Decora_1-Gang_v4 (Autodesk Fusion 360 design; units mm, degrees)
Autodesk Fusion 360 part; units mm, degrees
note: some values were not read from the file. Chosen so that the rebuilt part matches the saved one: which bodies a step acts on; which face or edge a step refers to; which pieces of a blend or face edit are solid. Set by a fixed rule: which sketch regions a step uses.
sketch "Sketch1" plane through (0, 0, 0) normal (0, 0, 1) x (1, 0, 0)
  line L0 (0, 0) -> (79.2, 0)
  line L1 (79.2, 0) -> (79.2, 123.8)
  line L2 (79.2, 123.8) -> (0, 123.8)
  line L3 (0, 123.8) -> (0, 0)
  line L4 (25, 95.3) -> (54.2, 95.3)
  line L5 (56.2, 93.3) -> (56.2, 30.5)
  line L6 (54.2, 28.5) -> (25, 28.5)
  line L7 (23, 30.5) -> (23, 93.3)
  line L8 (39.6, 28.5) -> (39.6, 95.3)
  line L9 (23, 61.9) -> (39.6, 61.9)
  line L10 (39.6, 0) -> (39.6, 123.8)
  line L11 (56.2, 61.9) -> (39.6, 61.9)
  circle A0 centre (39.6, 13.5) radius 3.5
  line L12 (36.1, 13.4847) -> (43.1, 13.4847)
  circle A1 centre (39.6, 110.3) radius 3.5
  circle A2 centre (39.6, 110.3) radius 1.5
  circle A3 centre (39.6, 13.5) radius 1.5
  line L13 (79.2, 61.9) -> (0, 61.9)
  line L14 (39.6, 106.8) -> (39.6, 113.8)
  arc A4 (23, 30.5) -> (25, 28.5) centre (25, 30.5) ccw
  arc A5 (54.2, 28.5) -> (56.2, 30.5) centre (54.2, 30.5) ccw
  arc A6 (56.2, 93.3) -> (54.2, 95.3) centre (54.2, 93.3) ccw
  arc A7 (25, 95.3) -> (23, 93.3) centre (25, 93.3) ccw
  point P0 (56.2, 95.3)
  point P1 (56.2, 28.5)
  point P2 (23, 28.5)
  dimension "d1" = 123.8
  dimension "d2" = 79.2
  dimension "d3" = 48.4
  dimension "d4" = 48.4
  dimension "d5" = 7
  dimension "d6" = 7
  dimension "d7" = 3
  dimension "d8" = 3
  dimension "d9" = 33.2
  dimension "d10" = 66.8
  dimension "d11" = 33.2
  dimension "d31" = 2
  dimension "d32" = 2
  dimension "d33" = 2
  dimension "d34" = 2
  constraint horizontal L0
  constraint vertical L1
  constraint horizontal L2
  constraint vertical L3
  constraint coincident L0.start L3.end
  constraint horizontal L4
  constraint vertical L5
  constraint horizontal L6
  constraint vertical L7
  constraint midpoint L0 L10.start
  constraint midpoint L2 L10.end
  constraint perpendicular L1 L11
  constraint collinear L8 L10
  constraint collinear L9 L11
  constraint coincident L10 A0.centre
  constraint coincident A0 L12.start
  constraint coincident A0 L12.end
  constraint perpendicular L10 L12
  constraint concentric A1 A2
  constraint concentric A0 A3
  constraint coincident L8 L9.end
  constraint midpoint L1 L13.start
  constraint midpoint L3 L13.end
  constraint collinear L11 L13
  constraint coincident A1 L14.start
  constraint coincident A1 L14.end
  constraint parallel L10 L14
  constraint midpoint A1.centre L14
  constraint collinear L10 L14
  constraint coincident L6 L8.start
  constraint coincident L7 L9.start
  constraint coincident P2 L6
  constraint coincident P2 L7
  constraint tangent L6 A4
  constraint tangent L7 A4
  constraint coincident L5 L11.start
  constraint coincident P1 L5
  constraint coincident P1 L6
  constraint tangent L5 A5
  constraint tangent L6 A5
  constraint coincident L4 L8.end
  constraint coincident P0 L4
  constraint coincident P0 L5
  constraint tangent L4 A6
  constraint tangent L5 A6
  constraint tangent L4 A7
  constraint tangent L7 A7
  constraint midpoint L7 L9.start
  constraint midpoint L6 L8.start
  constraint coincident L8.start L10
  measures "d1" distance of L0.end L1.end
  measures "d2" distance of L0.start L0.end
  measures "d3" vertical distance of L9.start A0.centre
  measures "d4" vertical distance of L11.start A1.centre
  measures "d5" diameter of A0
  measures "d6" diameter of A1
  measures "d7" diameter of A2
  measures "d8" diameter of A3
  measures "d9" distance of P1 P2
  measures "d10" distance of P0 P1
  measures "d11" distance of P1 P2
  measures "d31" radius of A4
  measures "d32" radius of A5
  measures "d33" radius of A6
  measures "d34" radius of A7
extrude "Extrude1" add sketch "Sketch1" along normal blind 6.4 contours L0 L3 L6 L7 L10 A0 L13 A4 | L0 L1 L5 L6 L10 A0 L13 A5 | L2 L3 L4 L7 L10 A1 L13 A7 | L10 A0 L12 A3 | L10 A0 L12 A3 | L1 L2 L4 L5 L10 A1 L13 A6 | L10 A0 L12 A3 | L10 A0 L12 A3 | L10 A1 A2 L14 | L10 A1 A2 L14 makes body 1
chamfer "Chamfer1" distance 3.5 angle 45 8 edges at (59.4, 123.8, 6.4) (19.8, 123.8, 6.4) (0, 92.85, 6.4) (0, 30.95, 6.4) (19.8, 0, 6.4) (59.4, 0, 6.4) (79.2, 30.95, 6.4) (79.2, 92.85, 6.4) on bodies 1
shell "Shell1" thickness 1.6 removed faces 1 at (7.6667, 51.4333, 0) on bodies 1
move_face "OffsetFaces1" offset -3.8 1 faces at (21.9333, 72.3667, 0) on bodies 1
move_face "OffsetFaces2" offset -4.8 1 faces at (41.9689, 109.3301, 0) on bodies 1
move_face "OffsetFaces3" offset -4.8 1 faces at (42.1495, 13.7285, 0) on bodies 1
chamfer "Chamfer2" distance 2 distance2 1.5 1 edges at (38.2015, 14.0424, 6.4) measured on face at (10, 51.4333, 6.4) on bodies 1
chamfer "Chamfer3" distance 2 distance2 1.5 1 edges at (38.2015, 110.8424, 6.4) measured on face at (10, 51.4333, 6.4) on bodies 1
sketch "Sketch2" plane through (0, 0, 6.4) normal (0, 0, 1) x (-1, 0, 0)
  circle A0 centre (-39.6, -13.5) radius 3.5
  arc A1 (-56.2, -93.3) -> (-54.2, -95.3) centre (-54.2, -93.3) ccw
  line L0 (-56.2, -93.3) -> (-56.2, -30.5)
  arc A2 (-54.2, -28.5) -> (-56.2, -30.5) centre (-54.2, -30.5) ccw
  line L1 (-54.2, -28.5) -> (-25, -28.5)
  arc A3 (-23, -30.5) -> (-25, -28.5) centre (-25, -30.5) ccw
  line L2 (-23, -30.5) -> (-23, -93.3)
  arc A4 (-25, -95.3) -> (-23, -93.3) centre (-25, -93.3) ccw
  line L3 (-25, -95.3) -> (-54.2, -95.3)
  line L4 (-3.5, -120.3) -> (-3.5, -3.5)
  line L5 (-3.5, -3.5) -> (-75.7, -3.5)
  line L6 (-75.7, -3.5) -> (-75.7, -120.3)
  line L7 (-75.7, -120.3) -> (-3.5, -120.3)
  circle A5 centre (-39.6, -110.3) radius 3.5
  line L8 (-39.6, -113.8) -> (-75.7, -113.8)
  point P0 (-39.6, -113.8)
  constraint coincident P0 L8.start
  constraint coincident L6 L8.end
  constraint tangent A5 L8
  constraint perpendicular L6 L8
split "Split1" by curves path "Sketch2" along L8 bodies 1 makes body 2 at (10, 49.2667, 6.4)
extrude "Extrude2" cut 3 faces at (63.4458, 113.8, 5.8667) (15.7542, 113.8, 5.8667) (76.8667, 113.8, 4.4791) along direction (0, -1, 0) blind 3 on bodies 2 bodies 2
move_face "MoveFace1" by (0, -3, 0) 3 faces at (15.7542, 113.8, 5.8667) (63.4458, 113.8, 5.8667) (76.8667, 113.8, 4.4791) on bodies 1
combine "Combine1" operation add target body 1 tool bodies 2
delete_face "DeleteFace17" 1 faces at (40.5261, 110.8, 6.2307) on bodies 1
sketch "Sketch3" plane through (0, 0, 6.4) normal (0, 0, 1) x (-1, 0, 0)
  line L0 (-39.6, -113.8) -> (-75.7, -113.8)
  line L1 (-75.7, -120.3) -> (-75.7, -3.5)
  line L2 (-39.6, -114.8) -> (-75.7, -114.8)
  line L3 (-39.6, -114.8) -> (-10.4528, -114.3)
  line L4 (-4.5, -120.3) -> (-10.4528, -114.3)
  point P0 (-39.6, -113.8)
  dimension "d37" = 1
  constraint coincident L1 L2.end
  measures "d37" distance of P0 L2.start
split "Split2" by curves path "Sketch3" along L4 L3 L2 bodies 1 makes body 3 at (10, 51.4333, 6.4)
delete_face "DeleteFace18" 2 faces at (63.4458, 114.8, 5.8667) (76.8667, 114.8, 4.4791) on bodies 3
move_face "MoveFace2" by (0.0172, -0.9999, 0) 1 faces at (53.73, 115.0424, 5.8667) on bodies 3
move_face "MoveFace3" by (0.0086, -0.4999, 0) 1 faces at (42.0019, 113.8411, 5.3332) on bodies 3
delete_face "DeleteFace19" 1 faces at (1.5092, 122.6333, 4.0667) on bodies 3
move_face "MoveFace4" by (0.0343, -1.9997, 0) 1 faces at (64.0298, 113.7189, 5.8667) on bodies 3
move_face "MoveFace5" by (0.4999, 0.0086, 0) 1 faces at (3.7575, 121.0484, 4.4791) on bodies 3
move_face "MoveFace6" by (0.0086, -0.4999, 0) 2 faces at (64.558, 111.7276, 5.8667) (21.6547, 110.9916, 5.8667) on bodies 3
named bodies: "decora_1_gang_chopped"
